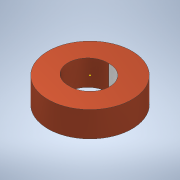
# Autodesk Inventor part: bobina_sin_numero
Saved by Autodesk Inventor 2020 (Build 240168000, 168)
## iProperties
Created: 2023-02-14
Part Number: bobina_sin_numero
Material: Generic
Document SubType Name: Modeling
Designer: General
Density: 1 g/cm^3
Appearance: Default
Author: General
Autodesk Inventor part; units mm, degrees
ref_plane "YZ Plane" through (0, 0, 0) normal (1, 0, 0) x (0, 1, 0)
ref_plane "XZ Plane" through (0, 0, 0) normal (0, 1, 0) x (-1, 0, 0)
ref_plane "XY Plane" through (0, 0, 0) normal (0, 0, 1) x (1, 0, 0)
sketch "Sketch1" plane through (0, 0, 0) normal (0, 1, 0) x (-1, 0, 0)
  circle A0 centre (0, 0) radius 48
  dimension "d0" = 96
  constraints: 1 centre point, 1 coincident
  measures "d0" diameter of A0
extrude "Extrusion1" add sketch "Sketch1" along normal blind 29.1
sketch "Sketch2" plane through (0, 29.1, 0) normal (0, 1, 0) x (1, 0, 0)
  point P0 (0, 0)
  point P1 (-2.5528, 0.0324)
hole "Hole1" at (-2.5528, 29.1, -0.0324) direction (0, -1, 0) diameter 45 end through all
sketch "Sketch3" plane through (0, 29.1, 0) normal (0, 1, 0) x (1, 0, 0)
  point P0 (0, 0)
sketch "Sketch4" plane through (0, 29.1, 0) normal (0, 1, 0) x (1, 0, 0)
  point P0 (0, 0)
hole "Hole2" at (0, 29.1, 0) direction (0, -1, 0) diameter 45 end through all
body "Solid1"
